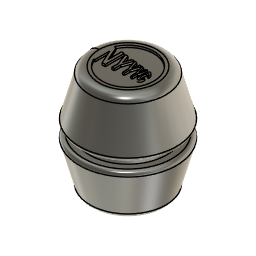
NYYYC CW v2 (Autodesk Fusion 360 design; units mm, degrees)
Autodesk Fusion 360 part; units mm, degrees
sketch "Sketch1" plane through (0, 0, 0) normal (1, 0, 0) x (0, 1, 0)
  line L0 (0, 0) -> (0, 16)
  line L1 (0, 16) -> (-6.9222, 16)
  line L2 (-9.0732, 14.2618) -> (-11.6071, 2.4599)
  line L3 (0, 0) -> (0, 2)
  line L4 (-10.6294, 1.25) -> (-9.2059, 1.25)
  line L5 (-9.2059, 1.25) -> (-9.2059, 0)
  arc A0 (-6.9222, 16) -> (-9.0732, 14.2618) centre (-6.9222, 13.8) ccw
  arc A1 (-11.6071, 2.4599) -> (-10.6294, 1.25) centre (-10.6294, 2.25) ccw
  line L6 (0, -16) -> (-6.9222, -16)
  arc A2 (-9.0732, -14.2618) -> (-6.9222, -16) centre (-6.9222, -13.8) ccw
  line L7 (-9.0732, -14.2618) -> (-11.6071, -2.4599)
  arc A3 (-10.6294, -1.25) -> (-11.6071, -2.4599) centre (-10.6294, -2.25) ccw
  line L8 (-10.6294, -1.25) -> (-9.2059, -1.25)
  line L9 (-9.2059, -1.25) -> (-9.2059, 0)
  line L10 (0, 0) -> (0, -16)
  point P0 (-8.7, 16)
  point P1 (-11.8669, 1.25)
  dimension "d1" = 16
  dimension "d2" = 8.7
  dimension "d4" = 2
  dimension "d6" = 2.2
  dimension "d7" = 1
  constraint coincident L0.start L3.start
  constraint vertical L0
  constraint perpendicular L0 L1
  constraint coincident L0 L3.end
  constraint coincident L2 P1
  constraint perpendicular L4 L5
  constraint coincident P0 L1
  constraint coincident P0 L2
  constraint tangent L1 A0
  constraint tangent L2 A0
  constraint coincident P1 L4
  constraint tangent L2 A1
  constraint tangent L4 A1
  measures "d1" distance of L0.start L0.end
  measures "d2" distance of L0.end P0
  measures "d4" distance of L0.start L3.end
  measures "d6" radius of A0
  measures "d7" radius of A1
revolve "Revolve1" add sketch "Sketch1" angle 360 about axis through (0, 0, 0) along (0, 0, 1)
scale "Scale1" factors (1.25, 1.25, 1) about (0, -9.2059, -1.25) bodies 1
sketch "Sketch2" plane through (0, 0, 16) normal (0, 0, 1) x (-1, 0, 0)
  circle A0 centre (0, -2.3015) radius 7.7362
  line L0 (7.1069, -5.3578) -> (6.56, -5.3)
  line L1 (6.56, -5.3) -> (4.7107, -1.0806)
  line L2 (4.7107, -1.0806) -> (4.7107, -5.0868)
  line L3 (4.7107, -5.0868) -> (3.8849, -4.9995)
  line L4 (3.8849, -4.9995) -> (3.8849, 0.5959)
  line L5 (3.8849, 0.5959) -> (4.77, 0.6863)
  line L6 (4.77, 0.6863) -> (6.6755, -3.4964)
  line L7 (6.6755, -3.4964) -> (6.6755, 0.8808)
  line L8 (6.6755, 0.8808) -> (7.0347, 0.9174)
  line L9 (3.4376, -4.9444) -> (2.1537, -1.5649)
  line L10 (2.1537, -1.5649) -> (2.1537, 0.3959)
  line L11 (2.1537, 0.3959) -> (1.4387, 0.3173)
  line L12 (1.4387, 0.3173) -> (1.4387, -1.5497)
  line L13 (1.4387, -1.5497) -> (0.3795, -4.6014)
  line L14 (0.3795, -4.6014) -> (1.1212, -4.6826)
  line L15 (1.1212, -4.6826) -> (1.7732, -2.5404)
  line L16 (3.4376, -4.9444) -> (2.5036, -4.8401)
  line L17 (2.5036, -4.8401) -> (1.7732, -2.5404)
  line L18 (0.2738, -4.5899) -> (-0.446, -4.5111)
  line L19 (-0.446, -4.5111) -> (-1.0015, -2.4871)
  line L20 (-1.0015, -2.4871) -> (-1.5087, -4.3891)
  line L21 (-1.5087, -4.3891) -> (-2.0913, -4.3254)
  line L22 (-2.0913, -4.3254) -> (-1.2559, -1.6387)
  line L23 (-1.2559, -1.6387) -> (-1.2559, 0.0121)
  line L24 (-1.2559, 0.0121) -> (-0.7119, 0.0736)
  line L25 (-0.7119, 0.0736) -> (-0.7119, -1.638)
  line L26 (-0.7119, -1.638) -> (0.2738, -4.5899)
  line L27 (-2.168, -4.3153) -> (-2.7331, -4.2568)
  line L28 (-2.7331, -4.2568) -> (-3.1751, -2.4683)
  line L29 (-3.1751, -2.4683) -> (-3.5825, -4.169)
  line L30 (-3.5825, -4.169) -> (-4.049, -4.1208)
  line L31 (-4.049, -4.1208) -> (-3.3788, -1.6981)
  line L32 (-3.3788, -1.6981) -> (-3.3788, -0.2213)
  line L33 (-3.3788, -0.2213) -> (-2.9424, -0.1725)
  line L34 (-2.9424, -0.1725) -> (-2.9424, -1.6981)
  line L35 (-2.9424, -1.6981) -> (-2.168, -4.3153)
  line L36 (-5.3424, -2.7778) -> (-5.6816, -2.7676)
  line L37 (-5.351, -1.6356) -> (-5.6747, -1.6437)
  spline S0 degree 5 poles (-4.6865, -3.0795) (-4.6776, -3.0458) (-4.6607, -2.9785) (-4.6385, -2.8774) (-4.6148, -2.7421) (-4.5942, -2.5717) (-4.5816, -2.3994) (-4.5764, -2.2243) (-4.5782, -2.0461) (-4.5876, -1.8649) (-4.6052, -1.6813) (-4.6266, -1.5328) (-4.6474, -1.4208) (-4.6633, -1.3458) (-4.6718, -1.3082) knots 0 0 0 0 0 0 0.1 0.2 0.3 0.4 0.5 0.6 0.7 0.8 0.9 1 1 1 1 1 1
  line L38 (-4.7332, -3.2552) -> (-4.6398, -2.9037)
  ellipse E0 centre (-4.996, -2.8015) end of major axis (-4.996, -3.4185) minor radius 0.3467 (-5.3424, -2.7778) -> (-4.6865, -3.0795) ccw
  line L39 (-4.6301, -1.4925) -> (-4.7135, -1.124)
  ellipse E1 centre (-4.9904, -1.623) end of major axis (-4.9904, -0.9507) minor radius 0.3606 (-4.64, -1.4644) -> (-4.6401, -1.4641) ccw
  ellipse E2 centre (-4.9904, -1.623) end of major axis (-4.9904, -0.9507) minor radius 0.3606 (-4.6718, -1.3082) -> (-5.351, -1.6356) ccw
  spline S1 degree 5 poles (-5.6816, -2.7676) (-5.6769, -2.8751) (-5.6613, -3.0793) (-5.6186, -3.3539) (-5.5231, -3.656) (-5.3422, -3.9239) (-5.1117, -4.0744) (-4.8528, -4.0971) (-4.6121, -3.9695) (-4.4179, -3.6897) (-4.2797, -3.2761) (-4.1979, -2.7614) (-4.1685, -2.1895) (-4.1898, -1.6122) (-4.2673, -1.0855) (-4.4074, -0.6617) (-4.6087, -0.3802) (-4.8584, -0.2625) (-5.118, -0.2966) (-5.3322, -0.4442) (-5.4924, -0.7051) (-5.5815, -1.0114) (-5.6331, -1.3027) (-5.6618, -1.5253) (-5.6747, -1.6437) knots 0 0 0 0 0 0 0.05 0.1 0.15 0.2 0.25 0.3 0.35 0.4 0.45 0.5 0.55 0.6 0.65 0.7 0.75 0.8 0.85 0.9 0.95 1 1 1 1 1 1
  line L40 (-5.1781, -4.0795) -> (-4.6837, -4.0587)
  line L41 (-4.6811, -0.3016) -> (-5.1651, -0.286)
  line L42 (-5.5892, -0.861) -> (-5.7602, -2.4264)
  point P0 (-4.5782, -2.2316)
  point P1 (-4.9309, -4.0691)
  point P2 (-4.1816, -2.2244)
  point P3 (-4.9231, -0.2938)
  constraint coincident A0 L0.start
  constraint vertical L2
  constraint parallel L0 L3
  constraint parallel L2 L4
  constraint parallel L4 L7
  constraint coincident A0 L8.end
  constraint parallel L5 L8
  constraint vertical L10
  constraint parallel L10 L12
  constraint parallel L14 L18
  constraint parallel L18 L21
  constraint vertical L23
  constraint parallel L23 L25
  constraint parallel L27 L30
  constraint vertical L32
  constraint parallel L32 L34
  constraint coincident S0.end E1
  constraint midpoint S0.start L38
  constraint midpoint S0.end L39
  constraint concentric E1 E2
  constraint midpoint P1 L40
  constraint midpoint P3 L41
  constraint midpoint L37.end L42
extrude "Extrude1" cut sketch "Sketch2" against normal blind 0.6 contours A0 L0 L1 L2 L3 L4 L5 L6 L7 L8 picked at (0.1488, 1.9402)
sketch "Sketch3" plane through (0, 0, -16) normal (0, 0, -1) x (1, 0, 0)
  arc A0 (-8.6528, -2.3015) -> (0, 6.3513) centre (0, -2.3015) ccw
  arc A1 (0, 6.3513) -> (-8.6528, -2.3015) centre (0, -2.3015) ccw
  line L0 (-0.7119, -1.638) -> (0.2738, -4.5899)
  ellipse E0 centre (-4.996, -2.8015) end of major axis (-4.996, -3.4185) minor radius 0.3467 (-5.3424, -2.7778) -> (-4.6865, -3.0795) ccw
  line L1 (4.77, 0.6863) -> (6.6755, -3.4964)
  line L2 (-1.2559, -1.6387) -> (-1.2559, 0.0121)
  line L3 (3.4376, -4.9444) -> (2.5036, -4.8401)
  line L4 (-2.0913, -4.3254) -> (-1.2559, -1.6387)
  circle A2 centre (0, -2.3015) radius 7.7362
  line L5 (2.1537, 0.3959) -> (1.4387, 0.3173)
  line L6 (-4.049, -4.1208) -> (-3.3788, -1.6981)
  line L7 (-3.3788, -0.2213) -> (-2.9424, -0.1725)
  line L8 (6.6755, -3.4964) -> (6.6755, 0.8808)
  line L9 (-2.9424, -1.6981) -> (-2.168, -4.3153)
  line L10 (2.5036, -4.8401) -> (1.7732, -2.5404)
  line L11 (2.1537, -1.5649) -> (2.1537, 0.3959)
  ellipse E1 centre (-4.9904, -1.623) end of major axis (-4.9904, -0.9507) minor radius 0.3606 (-4.6718, -1.3082) -> (-5.351, -1.6356) ccw
  spline S0 degree 5 poles (-5.6816, -2.7676) (-5.6769, -2.8751) (-5.6613, -3.0793) (-5.6186, -3.3539) (-5.5231, -3.656) (-5.3422, -3.9239) (-5.1117, -4.0744) (-4.8528, -4.0971) (-4.6121, -3.9695) (-4.4179, -3.6897) (-4.2797, -3.2761) (-4.1979, -2.7614) (-4.1685, -2.1895) (-4.1898, -1.6122) (-4.2673, -1.0855) (-4.4074, -0.6617) (-4.6087, -0.3802) (-4.8584, -0.2625) (-5.118, -0.2966) (-5.3322, -0.4442) (-5.4924, -0.7051) (-5.5815, -1.0114) (-5.6331, -1.3027) (-5.6618, -1.5253) (-5.6747, -1.6437) knots 0 0 0 0 0 0 0.05 0.1 0.15 0.2 0.25 0.3 0.35 0.4 0.45 0.5 0.55 0.6 0.65 0.7 0.75 0.8 0.85 0.9 0.95 1 1 1 1 1 1
  line L12 (-5.1781, -4.0795) -> (-4.6837, -4.0587)
  line L13 (-4.6811, -0.3016) -> (-5.1651, -0.286)
  line L14 (-5.5892, -0.861) -> (-5.7602, -2.4264)
  line L15 (6.6755, 0.8808) -> (7.0347, 0.9174)
  line L16 (-2.168, -4.3153) -> (-2.7331, -4.2568)
  line L17 (-3.3788, -1.6981) -> (-3.3788, -0.2213)
  line L18 (3.8849, -4.9995) -> (3.8849, 0.5959)
  line L19 (3.4376, -4.9444) -> (2.1537, -1.5649)
  line L20 (7.1069, -5.3578) -> (6.56, -5.3)
  line L21 (-0.7119, 0.0736) -> (-0.7119, -1.638)
  line L22 (0.3795, -4.6014) -> (1.1212, -4.6826)
  line L23 (0.2738, -4.5899) -> (-0.446, -4.5111)
  line L24 (4.7107, -5.0868) -> (3.8849, -4.9995)
  line L25 (4.7107, -1.0806) -> (4.7107, -5.0868)
  line L26 (-0.446, -4.5111) -> (-1.0015, -2.4871)
  line L27 (-1.2559, 0.0121) -> (-0.7119, 0.0736)
  line L28 (-3.5825, -4.169) -> (-4.049, -4.1208)
  line L29 (1.4387, 0.3173) -> (1.4387, -1.5497)
  line L30 (-3.1751, -2.4683) -> (-3.5825, -4.169)
  ellipse E2 centre (-4.9904, -1.623) end of major axis (-4.9904, -0.9507) minor radius 0.3606 (-4.64, -1.4644) -> (-4.6401, -1.4641) ccw
  line L31 (6.56, -5.3) -> (4.7107, -1.0806)
  line L32 (-2.7331, -4.2568) -> (-3.1751, -2.4683)
  line L33 (-5.3424, -2.7778) -> (-5.6816, -2.7676)
  line L34 (3.8849, 0.5959) -> (4.77, 0.6863)
  line L35 (1.1212, -4.6826) -> (1.7732, -2.5404)
  line L36 (1.4387, -1.5497) -> (0.3795, -4.6014)
  line L37 (-2.9424, -0.1725) -> (-2.9424, -1.6981)
  spline S1 degree 5 poles (-4.6865, -3.0795) (-4.6776, -3.0458) (-4.6607, -2.9785) (-4.6385, -2.8774) (-4.6148, -2.7421) (-4.5942, -2.5717) (-4.5816, -2.3994) (-4.5764, -2.2243) (-4.5782, -2.0461) (-4.5876, -1.8649) (-4.6052, -1.6813) (-4.6266, -1.5328) (-4.6474, -1.4208) (-4.6633, -1.3458) (-4.6718, -1.3082) knots 0 0 0 0 0 0 0.1 0.2 0.3 0.4 0.5 0.6 0.7 0.8 0.9 1 1 1 1 1 1
  line L38 (-4.7332, -3.2552) -> (-4.6398, -2.9037)
  line L39 (-4.6301, -1.4925) -> (-4.7135, -1.124)
  line L40 (-5.351, -1.6356) -> (-5.6747, -1.6437)
  line L41 (-1.5087, -4.3891) -> (-2.0913, -4.3254)
  line L42 (-1.0015, -2.4871) -> (-1.5087, -4.3891)
  point P0 (-4.1816, -2.2244)
  point P1 (-4.9309, -4.0691)
  point P2 (-4.9231, -0.2938)
  point P3 (-4.5782, -2.2316)
  constraint coincident L20.start A2
  constraint vertical L25
  constraint parallel L20 L24
  constraint parallel L18 L25
  constraint parallel L8 L18
  constraint coincident L15.end A2
  constraint parallel L15 L34
  constraint vertical L11
  constraint parallel L11 L29
  constraint parallel L22 L23
  constraint parallel L23 L41
  constraint vertical L2
  constraint parallel L2 L21
  constraint parallel L16 L28
  constraint vertical L17
  constraint parallel L17 L37
  constraint coincident S1.end E2
  constraint midpoint S1.start L38
  constraint midpoint S1.end L39
  constraint concentric E1 E2
  constraint midpoint P1 L12
  constraint midpoint P2 L13
  constraint midpoint S0.end L14
extrude "Extrude2" cut sketch "Sketch3" against normal blind 0.6 contours L1 A2 L8 L15 L18 L20 L24 L25 L31 L34 picked at (0.1488, 1.9402)
